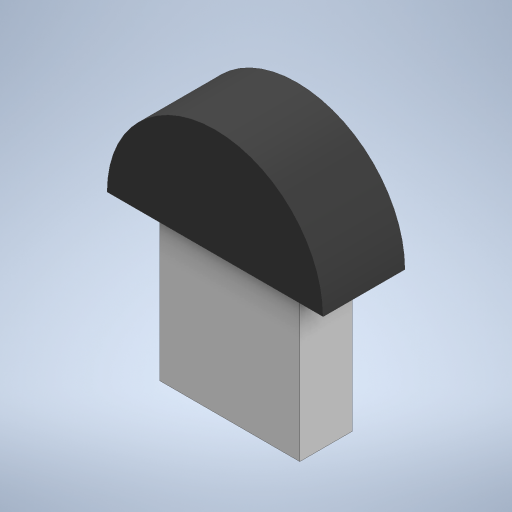
# Autodesk Inventor part: Mic
Saved by Autodesk Inventor 2023.1 (Build 271208000, 208)
## iProperties
Created: 2022-08-09
Part Number: Mic
Material: 일반
Document SubType Name: Modeling
Designer: fly01
Density: 1 g/cm^3
Appearance: 기본값
Author: fly01
Autodesk Inventor part; units mm, degrees
ref_plane "YZ Plane" through (0, 0, 0) normal (1, 0, 0) x (0, 1, 0)
ref_plane "XZ Plane" through (0, 0, 0) normal (0, 1, 0) x (-1, 0, 0)
ref_plane "XY Plane" through (0, 0, 0) normal (0, 0, 1) x (1, 0, 0)
sketch "스케치1" plane through (0, 0, 0) normal (0, 0, 1) x (1, 0, 0)
  line L0 (-9.25, 0) -> (9.25, 0)
  arc A0 (9.25, 0) -> (-9.25, 0) centre (0, 0) ccw
  line L1 (0, 9.25) -> (0, 0) construction
  line L2 (-6, 0) -> (6, 0)
  line L3 (6, 0) -> (6, -13)
  line L4 (6, -13) -> (-6, -13)
  line L5 (-6, -13) -> (-6, 0)
  dimension "d0" = 18.5
  dimension "d1" = 9.25
  dimension "d2" = 12
  dimension "d3" = 13
  constraints: 12 end point, 3 point on circle, 2 horizontal, 2 midpoint, 2 parallel, 2 perpendicular, 1 centre point, 1 coincident, 1 point on line
  measures "d0" distance of L0.start L0.end
  measures "d1" distance of L1.start L1.end
  measures "d2" distance of L3.end L4.end
  measures "d3" distance of L2.end L3.end
extrude "돌출1" add sketch "스케치1" along normal mid plane 7 contours A0 L0
extrude "돌출2" add sketch "스케치1" along normal mid plane 4.5 contours L0 L3 L4 L5
